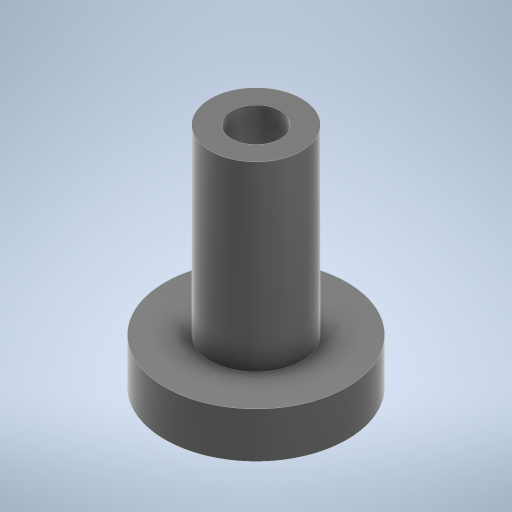
# Autodesk Inventor part: D3260-12120LB
Saved by Autodesk Inventor 2024.2 (Build 282272000, 272)
## iProperties
Created: 2024-01-05
Part Number: D3260-12120LB
Material: Acetal Resin, Black
Document SubType Name: Modeling
Designer: Masato Kubotera
Density: 1.425 g/cm^3
Appearance: Smooth - Black
Catalog Web Link: https://www.hirosugi-net.co.jp/shop/g/g103787/
Vendor: HIROSUGI
Mass: 0.136345 g
Surface Area: 1.42942 cm^2
Volume: 0.0486947 cm^3
Author: Masato Kubotera
Autodesk Inventor part; units mm, degrees
ref_plane "YZ Plane" through (0, 0, 0) normal (1, 0, 0) x (0, 1, 0)
ref_plane "XZ Plane" through (0, 0, 0) normal (0, 1, 0) x (-1, 0, 0)
ref_plane "XY Plane" through (0, 0, 0) normal (0, 0, 1) x (1, 0, 0)
sketch "Sketch1" plane through (0, 0, 0) normal (0, 1, 0) x (-1, 0, 0)
  line L0 (0, 0) -> (0, 15)
  line L1 (-1.6, 15) -> (-1.6, 0)
  line L2 (-1.6, 0) -> (-6, 0)
  line L3 (-6, 0) -> (-6, 3)
  line L4 (-6, 3) -> (-3, 3)
  line L5 (-3, 3) -> (-3, 15)
  line L6 (-3, 15) -> (-1.6, 15)
  dimension "d0" = 3.2
  dimension "d1" = 6
  dimension "d2" = 12
  dimension "d3" = 3
  dimension "d4" = 12
  constraints: 14 end point, 3 horizontal, 3 vertical, 2 point on line, 1 perpendicular
  measures "d0" diameter of L1 L0
  measures "d1" diameter of L5 L0
  measures "d2" diameter of L3 L0
  measures "d3" distance of L2.end L3.end
  measures "d4" distance of L4.end L5.end
revolve "Revolution1" add sketch "Sketch1" angle 360 about axis through (0, 0, 0) along (0, 0, 1)
body "Solid1"
